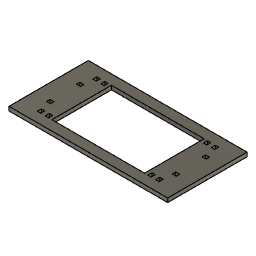
Test Base v4 (Autodesk Fusion 360 design; units mm, degrees)
Autodesk Fusion 360 part; units mm, degrees
sketch "Sketch1" plane through (0, 0, 0) normal (0, 0, 1) x (1, 0, 0) in component "Base"
  line L0 (120, 60) -> (-120, 60)
  line L1 (-120, 60) -> (-120, -60)
  line L2 (-120, -60) -> (120, -60)
  line L3 (120, -60) -> (120, 60)
  line L4 (120, 60) -> (-120, -60) construction
  line L5 (-120, 60) -> (120, -60) construction
  line L6 (-70, 45) -> (70, 45)
  line L7 (70, 45) -> (70, -45)
  line L8 (70, -45) -> (-70, -45)
  line L9 (-70, -45) -> (-70, 45)
  line L10 (-70, 45) -> (70, -45) construction
  line L11 (70, 45) -> (-70, -45) construction
  dimension "d1" = 240
  dimension "d2" = 120
  dimension "d3" = 90
  dimension "d6" = 140
  constraint horizontal L0
  constraint perpendicular L0 L1
  constraint parallel L0 L2
  constraint parallel L1 L3
  constraint coincident L4 origin
  constraint coincident L5 origin
  constraint horizontal L6
  constraint perpendicular L6 L7
  constraint parallel L6 L8
  constraint parallel L7 L9
  constraint coincident L10 origin
  constraint coincident L11 origin
  measures "d1" distance of L1.end L2.end
  measures "d2" distance of L0.end L1.end
  measures "d3" distance of L6.end L7.end
  measures "d6" distance of L7 L9
extrude "Extrude1" add sketch "Sketch1" along normal blind 6 in component "Base"
sketch "Sketch2" plane through (0, 0, 6) normal (0, 0, 1) x (-1, 0, 0) in component "Base"
  line L0 (-70, 45) -> (70, 45)
  line L1 (70, 45) -> (70, -45)
  line L2 (70, -45) -> (-70, -45)
  line L3 (-70, -45) -> (-70, 45)
  line L4 (-120, 60) -> (-120, -60)
  line L5 (-120, -60) -> (120, -60)
  line L6 (120, -60) -> (120, 60)
  line L7 (120, 60) -> (-120, 60)
  line L8 (70, 45) -> (92, 45) construction
  line L9 (92, 45) -> (92, 39) construction
  line L10 (92, 39) -> (70, 39) construction
  line L11 (70, 39) -> (70, 45) construction
  line L12 (92, 39) -> (87, 39)
  line L13 (87, 39) -> (87, 45)
  line L14 (87, 45) -> (92, 45)
  line L15 (92, 45) -> (92, 39)
  line L16 (70, 39) -> (75, 39) construction
  line L17 (75, 45) -> (75, 39) construction
  line L18 (75, 39) -> (80, 39)
  line L19 (80, 39) -> (80, 45)
  line L20 (80, 45) -> (75, 45)
  line L21 (75, 45) -> (75, 39)
  dimension "d15" = 6
  constraint horizontal L8
  constraint vertical L9
  constraint horizontal L10
  constraint vertical L11
  constraint coincident L0.end L1.start
  constraint horizontal L12
  constraint vertical L13
  constraint horizontal L14
  constraint vertical L15
  constraint coincident L8 L13.end
  constraint coincident L10 L16.end
  constraint coincident L8 L17.start
  constraint perpendicular L10 L17
  constraint horizontal L18
  constraint vertical L19
  constraint horizontal L20
  constraint vertical L21
  constraint coincident L8 L19.end
  measures "d15" distance of L8 L12
extrude "Extrude2" cut sketch "Sketch2" against normal blind 6 contours L12 L13 L14 L15 | L18 L19 L20 L21 in component "Base"
ref_plane "WorkPlane1" through (0, 0, 0) normal (1, 0, 0) x (0, 1, 0) in component "Base"
mirror "Mirror1" about plane through (0, 0, 0) normal (1, 0, 0) of "Extrude2" in component "Base"
ref_plane "WorkPlane2" through (0, 0, 0) normal (0, 1, 0) x (0, 0, 1) in component "Base"
mirror "Mirror2" about plane through (0, 0, 0) normal (0, 1, 0) of "Extrude2", "Mirror1" in component "Base"
sketch "Sketch3" plane through (0, 0, 0) normal (0, 0, -1) x (1, 0, 0) in component "Base"
  line L0 (87, -45) -> (87, -39)
  line L1 (87, -39) -> (92, -39)
  line L2 (92, -39) -> (92, -45)
  line L3 (92, -45) -> (87, -45)
  line L4 (75, -39) -> (80, -39)
  line L5 (80, -39) -> (80, -45)
  line L6 (80, -45) -> (75, -45)
  line L7 (75, -45) -> (75, -39)
  line L8 (-87, -39) -> (-87, -45)
  line L9 (-87, -45) -> (-92, -45)
  line L10 (-92, -45) -> (-92, -39)
  line L11 (-92, -39) -> (-87, -39)
  line L12 (-80, -39) -> (-75, -39)
  line L13 (-75, -39) -> (-75, -45)
  line L14 (-75, -45) -> (-80, -45)
  line L15 (-80, -45) -> (-80, -39)
  line L16 (87, 39) -> (87, 45)
  line L17 (87, 45) -> (92, 45)
  line L18 (92, 45) -> (92, 39)
  line L19 (92, 39) -> (87, 39)
  line L20 (80, 39) -> (75, 39)
  line L21 (75, 39) -> (75, 45)
  line L22 (75, 45) -> (80, 45)
  line L23 (80, 45) -> (80, 39)
  line L24 (-87, 45) -> (-87, 39)
  line L25 (-87, 39) -> (-92, 39)
  line L26 (-92, 39) -> (-92, 45)
  line L27 (-92, 45) -> (-87, 45)
  line L28 (-75, 39) -> (-80, 39)
  line L29 (-80, 39) -> (-80, 45)
  line L30 (-80, 45) -> (-75, 45)
  line L31 (-75, 45) -> (-75, 39)
  line L32 (-70, 45) -> (70, 45)
  line L33 (70, 45) -> (70, -45)
  line L34 (70, -45) -> (-70, -45)
  line L35 (-70, -45) -> (-70, 45)
  line L36 (120, -60) -> (120, 60)
  line L37 (120, 60) -> (-120, 60)
  line L38 (-120, 60) -> (-120, -60)
  line L39 (-120, -60) -> (120, -60)
  line L40 (-120, 0) -> (-70, 0) construction
  line L41 (-87, -39) -> (-87, 39) construction
  line L42 (-87, 0) -> (-87, -20) construction
  line L43 (-87, 0) -> (-87, -20) construction
  line L44 (-87, 0) -> (-93, 0) construction
  line L45 (-87, 0) -> (-92, 0) construction
  line L46 (-92, 0) -> (-92, -20) construction
  line L47 (-92, -20) -> (-87, -20) construction
  line L48 (-87, -20) -> (-87, 0) construction
  line L49 (-87, 0) -> (-91.9449, 0) construction
  line L50 (-91.9449, 20) -> (-87, 20) construction
  line L51 (-87, 20) -> (-87, 0) construction
  line L52 (-87, 0) -> (-92, 0) construction
  line L53 (-92, 0) -> (-92, 20) construction
  line L54 (-92, 20) -> (-87, 20) construction
  line L55 (-87, 20) -> (-87, 0) construction
  line L56 (-92, -20) -> (-98, -20)
  line L57 (-98, -20) -> (-98, -25)
  line L58 (-98, -25) -> (-92, -25)
  line L59 (-92, -25) -> (-92, -20)
  line L60 (-92, 20) -> (-98, 20)
  line L61 (-98, 20) -> (-98, 25)
  line L62 (-98, 25) -> (-92, 25)
  line L63 (-92, 25) -> (-92, 20)
  dimension "d16" = 5
  dimension "d17" = 20
  dimension "d18" = 20
  constraint midpoint L38 L40.start
  constraint midpoint L35 L40.end
  constraint coincident L8.start L11.end
  constraint coincident L24.end L25.start
  constraint midpoint L41 L42.start
  constraint coincident L41 L42.end
  constraint perpendicular L40 L42
  constraint coincident L40 L44.end
  constraint perpendicular L41 L44
  constraint horizontal L45
  constraint vertical L46
  constraint horizontal L47
  constraint vertical L48
  constraint horizontal L49
  constraint horizontal L50
  constraint vertical L51
  constraint horizontal L52
  constraint vertical L53
  constraint horizontal L54
  constraint vertical L55
  constraint horizontal L56
  constraint vertical L57
  constraint horizontal L58
  constraint vertical L59
  constraint horizontal L60
  constraint vertical L61
  constraint horizontal L62
  constraint vertical L63
  measures "d16" distance of L42.start L45.end
  measures "d17" distance of L42.start L42.end
  measures "d18" distance of L42.start L50.end
extrude "Extrude3" cut sketch "Sketch3" against normal blind 11 contours L56 L57 L58 L59 | L60 L61 L62 L63 in component "Base"
mirror "Mirror3" about plane through (0, 0, 0) normal (1, 0, 0) of "Extrude3" in component "Base"
component "Base" placed x (1, 0, 0) y (0, 1, 0) z (0, 0, 1) at (0, 0, 0)
